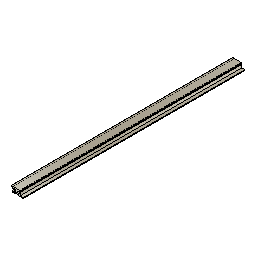
Tip Top Z Rails (Autodesk Fusion 360 design; units mm, degrees)
Autodesk Fusion 360 part; units mm, degrees
sketch "Sketch1" plane through (0, 0, 0) normal (0, 1, 0) x (1, 0, 0)
  circle A0 centre (0, 0) radius 2
  line L0 (-14, -4.7) -> (3.8, -4.7)
  line L1 (-14, -4.7) -> (-14, -3.54)
  line L2 (-14, -3.54) -> (-11.2, -3.54)
  line L3 (-11.2, -3.54) -> (-11.2, -1.54)
  line L4 (-11.2, -1.54) -> (-9.2, -1.54)
  line L5 (-9.2, -1.54) -> (-9.2, -2.54)
  line L6 (-9.2, -2.54) -> (-7.2, -2.54)
  line L7 (-7.2, -2.54) -> (-7.2, -1.54)
  line L8 (-7.2, -1.54) -> (-4.7, -1.54)
  line L9 (-4.7, -1.54) -> (-4.7, 2.46)
  line L10 (-4.7, 2.46) -> (-7.2, 2.46)
  line L11 (-7.2, 2.46) -> (-7.2, 3.46)
  line L12 (-7.2, 3.46) -> (-9.2, 3.46)
  line L13 (-9.2, 3.46) -> (-9.2, 2.46)
  line L14 (-9.2, 2.46) -> (-11.5, 2.46)
  line L15 (-11.5, 2.46) -> (-11.5, 5.3)
  line L16 (-11.5, 5.3) -> (-5, 5.3)
  line L17 (-5, 5.3) -> (-5, 4.3)
  line L18 (-5, 4.3) -> (0, 4.3)
  line L19 (0, 4.3) -> (0, 5.3)
  line L20 (0, 5.3) -> (9.5, 5.3)
  line L21 (9.5, 5.3) -> (9.5, 3.8)
  line L22 (9.5, 3.8) -> (3.5, 3.8)
  line L23 (3.8, -4.7) -> (3.8, -3.54)
  line L24 (3.8, -3.54) -> (1.5, -3.54)
  line L25 (1.5, -3.54) -> (1.5, -1.9)
  line L26 (1.5, -1.9) -> (3.5, -1.9)
  line L27 (3.5, -1.9) -> (3.5, 3.8)
  dimension "d1" = 4
  dimension "d2" = 17.8
  dimension "d3" = 2.8
  dimension "d4" = 5
  dimension "d5" = 1.16
  dimension "d6" = 2
  dimension "d7" = 2
  dimension "d8" = 2
  dimension "d9" = 1
  dimension "d10" = 4
  dimension "d11" = 2.5
  dimension "d12" = 1
  dimension "d13" = 1
  dimension "d15" = 2.5
  dimension "d17" = 6.5
  dimension "d18" = 1.16
  dimension "d21" = 1.5
  dimension "d22" = 9.5
  dimension "d23" = 3.8
  dimension "d25" = 6
  dimension "d26" = 10
  dimension "d27" = 1
  dimension "d28" = 2
  dimension "d29" = 1.64
  dimension "d30" = 3.5
  constraint coincident A0.centre origin
  constraint horizontal L0
  constraint perpendicular L0 L1
  constraint perpendicular L1 L2
  constraint perpendicular L0 L3
  constraint perpendicular L3 L4
  constraint perpendicular L0 L5
  constraint perpendicular L5 L6
  constraint perpendicular L6 L7
  constraint perpendicular L7 L8
  constraint perpendicular L6 L9
  constraint perpendicular L9 L10
  constraint perpendicular L6 L11
  constraint perpendicular L9 L12
  constraint perpendicular L6 L13
  constraint perpendicular L13 L14
  constraint perpendicular L14 L15
  constraint perpendicular L13 L16
  constraint perpendicular L16 L17
  constraint perpendicular L17 L18
  constraint perpendicular L18 L19
  constraint perpendicular L19 L20
  constraint perpendicular L18 L21
  constraint perpendicular L21 L22
  constraint perpendicular L0 L23
  constraint perpendicular L23 L24
  constraint perpendicular L24 L25
  constraint perpendicular L25 L26
  constraint perpendicular L26 L27
  constraint collinear L7 L11
  constraint collinear L5 L13
  constraint collinear L10 L14
  constraint collinear L16 L20
  constraint coincident L22.end L27.end
  measures "d1" diameter of A0
  measures "d2" distance of L0.start L0.end
  measures "d3" distance of L1.end L2.end
  measures "d4" distance of L17.end L18.end
  measures "d5" distance of L0.start L1.end
  measures "d6" distance of L3.end L4.end
  measures "d7" distance of L2.end L3.end
  measures "d8" distance of L5.end L6.end
  measures "d9" distance of L4.end L5.end
  measures "d10" distance of L8.end L9.end
  measures "d11" distance of L1 L15
  measures "d12" distance of L6.end L7.end
  measures "d13" distance of L10.end L11.end
  measures "d15" distance of L7.end L8.end
  measures "d17" distance of L15.end L16.end
  measures "d18" distance of L0.end L23.end
  measures "d21" distance of L20.end L21.end
  measures "d22" distance of L19.end L20.end
  measures "d23" distance of A0.centre L22
  measures "d25" distance of L21.end L22.end
  measures "d26" distance of L0 L20
  measures "d27" distance of L16.end L17.end
  measures "d28" distance of L25.end L26.end
  measures "d29" distance of L24.end L25.end
  measures "d30" distance of A0.centre L27
extrude "Extrude1" add sketch "Sketch1" along normal mid plane 426.72
equation "HP84 = 426.72 mm"
equation "d32 = HP84"
